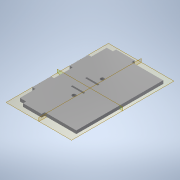
# Autodesk Inventor part: Plaat voor
Saved by Autodesk Inventor 2021 (Build 250183000, 183)
## iProperties
Manager: PJ / DCS
Company: Emmaüs Bovenbouw Aalter
Created: 2021-01-09
Part Number: Plaat voor
Material: S235
Catalog Web Link: http://emmausbovenbouw.op-weg.be/
Vendor: Emmaüsinstituut Bovenbouw Aalter
Document SubType Name: Modeling
Designer: Antho
Engineer: Declercq St.
Manufacturer: Standard
Standards Organization: Custom
Density: 7.86 g/cm^3
Appearance: Steel
Title: Algemene titel
Subject: Specifieke titel
Author: Antho
Keywords: Ruwe Ø xxxxx
Comments: Opmerking
Autodesk Inventor part; units mm, degrees
sketch "Sketch1" plane through (0, 0, 0) normal (0, 0, 1) x (1, 0, 0)
  line L0 (0, 2.8582) -> (0, -2.8582) construction
  line L1 (-5.7775, 0) -> (5.7775, 0) construction
  line L2 (-48, -75) -> (48, -75)
  line L3 (48, -75) -> (48, 75)
  line L4 (48, 75) -> (-48, 75)
  line L5 (-48, 75) -> (-48, -75)
  line L6 (-48, -75) -> (48, 75) construction
  line L7 (48, -75) -> (-48, 75) construction
  point P0 (0, 0)
  point P1 (0, 0)
  dimension "d0" = 96
  dimension "d1" = 150
  constraints: 16 end point, 4 midpoint, 2 horizontal, 2 parallel, 1 coincident, 1 perpendicular, 1 vertical
  measures "d0" distance of L4.end L3.end
  measures "d1" distance of L3.end L2.end
extrude "Extrusion1" add sketch "Sketch1" along normal blind 5
sketch "Sketch2" plane through (0, 0, 5) normal (0, 0, 1) x (1, 0, 0)
  line L0 (-48, 75) -> (-48, -75) projected
  line L1 (-48, 0) -> (-48, -15)
  line L2 (-48, -15) -> (-48, 15)
  line L3 (-48, 15) -> (-48, 45)
  line L4 (-48, 45) -> (-48, 75)
  line L5 (-48, -15) -> (-48, -45)
  line L6 (-48, -45) -> (-48, -75)
  line L7 (-48, -15) -> (-43, -15)
  line L8 (-43, -15) -> (-43, 15)
  line L9 (-43, 15) -> (-48, 15)
  line L10 (-48, 15) -> (-48, -15)
  line L11 (48, 75) -> (-48, 75) projected
  line L12 (-48, 45) -> (-43, 45)
  line L13 (-43, 45) -> (-43, 75)
  line L14 (-43, 75) -> (-48, 75)
  line L15 (-48, 75) -> (-48, 45)
  line L16 (-48, -45) -> (-43, -45)
  line L17 (-43, -45) -> (-43, -75)
  line L18 (-43, -75) -> (-48, -75)
  line L19 (-48, -75) -> (-48, -45)
  line L20 (-48, -75) -> (-33, -75)
  line L21 (-33, -75) -> (-33, -67)
  line L22 (-33, -67) -> (-48, -67)
  line L23 (-48, -67) -> (-48, -75)
  line L24 (-33, -75) -> (-3, -75)
  line L25 (-48, -75) -> (48, -75) projected
  line L26 (-3, -75) -> (27, -75)
  line L27 (-3, -75) -> (48, -75)
  line L28 (48, -75) -> (48, -67)
  line L29 (48, -67) -> (-3, -67)
  line L30 (-3, -67) -> (-3, -75)
  line L31 (-48, 75) -> (-33, 75)
  line L32 (-33, 75) -> (-33, 70)
  line L33 (-33, 70) -> (-48, 70)
  line L34 (-48, 70) -> (-48, 75)
  line L35 (48, -75) -> (48, 75) projected
  line L36 (-3, 75) -> (48, 75)
  line L37 (48, 75) -> (48, 70)
  line L38 (48, 70) -> (-3, 70)
  line L39 (-3, 70) -> (-3, 75)
  line L40 (-48, -75) -> (-33, -75)
  line L41 (-33, -75) -> (-33, -70)
  line L42 (-33, -70) -> (-48, -70)
  line L43 (-48, -70) -> (-48, -75)
  line L44 (-3, -75) -> (48, -75)
  line L45 (48, -75) -> (48, -70)
  line L46 (48, -70) -> (-3, -70)
  line L47 (-3, -70) -> (-3, -75)
  point P0 (0, 0)
  point P1 (-43, 70)
  point P2 (-33, 75)
  point P3 (-43, -67)
  point P4 (-43, -70)
  dimension "d4" = 15
  dimension "d5" = 30
  dimension "d6" = 30
  dimension "d7" = 30
  dimension "d8" = 30
  dimension "d9" = 5
  dimension "d10" = 15
  dimension "d12" = 30
  dimension "d13" = 30
  dimension "d14" = 51
  dimension "d15" = 5
  dimension "d18" = 15
  dimension "d23" = 8
  dimension "d24" = 5
  constraints: 88 end point, 18 parallel, 16 point on line, 9 horizontal, 9 perpendicular, 2 collinear, 1 midpoint
  measures "d4" distance of L1.start L1.end
  measures "d5" distance of L1.end L2.end
  measures "d6" distance of L2.end L3.end
  measures "d7" distance of L1.end L5.end
  measures "d8" distance of L5.end L0.end
  measures "d9" distance of L9.end L8.end
  measures "d10" distance of L22.end L21.end
  measures "d12" distance of L20.end L24.end
  measures "d13" distance of L24.end L26.end
  measures "d14" distance of L29.end L28.end
  measures "d15" distance of L31.end L32.end
  measures "d18" distance of L32.end L33.end
  measures "d23" distance of L20.end L21.end
  measures "d24" distance of L41.end L40.end
extrude "Extrusion2" cut sketch "Sketch2" against normal blind 8 contours L11 L13 L33 L0 | L33 L13 L12 L0 | L11 L32 L33 L13 | L9 L8 L7 L0 | L11 L35 L38 L39 | L16 L17 L22 L0 | L22 L17 L42 L0 | L28 L25 L30 L46 | L42 L17 L18 L0 | L42 L21 L20 L17
sketch "Sketch4" plane through (0, 0, 5) normal (0, 0, 1) x (1, 0, 0)
  line L0 (-43, 15) -> (-43, -15) projected
  line L1 (-43, 0) -> (-18, 0)
  line L2 (-18, 0) -> (-18, -12.8)
  line L3 (-18, -12.8) -> (2.5, -12.8)
  line L4 (2.5, -12.8) -> (2.5, -10.2)
  line L5 (2.5, -10.2) -> (-18, -10.2)
  line L6 (-18, 0) -> (-18, 12.8)
  line L7 (-18, 12.8) -> (2.5, 12.8)
  line L8 (2.5, 12.8) -> (2.5, 10.2)
  line L9 (2.5, 10.2) -> (-18, 10.2)
  circle A0 centre (-3, -22.8) radius 3
  circle A1 centre (-3, 22.8) radius 3
  point P0 (0, 0)
  dimension "d25" = 25
  dimension "d26" = 12.8
  dimension "d27" = 20.5
  dimension "d28" = 2.6
  dimension "d29" = 12.8
  dimension "d30" = 20.5
  dimension "d31" = 2.6
  dimension "d36" = 6
  dimension "d37" = 6
  dimension "d39" = 15
  dimension "d40" = 10
  dimension "d41" = 15
  dimension "d42" = 10
  constraints: 18 end point, 5 perpendicular, 5 point on line, 2 centre point, 1 horizontal, 1 midpoint
  measures "d25" distance of L1.start L1.end
  measures "d26" distance of L1.end L2.end
  measures "d27" distance of L2.end L3.end
  measures "d28" distance of L3.end L4.end
  measures "d29" distance of L1.end L6.end
  measures "d30" distance of L6.end L7.end
  measures "d31" distance of L7.end L8.end
  measures "d36" diameter of A0
  measures "d37" diameter of A1
  measures "d39" distance from line of L6 A1.centre
  measures "d40" distance from line of L7 A1.centre
  measures "d41" distance from line of L2 A0.centre
  measures "d42" distance from line of L3 A0.centre
extrude "Extrusion4" cut sketch "Sketch4" against normal blind 10
body "Solid1"
